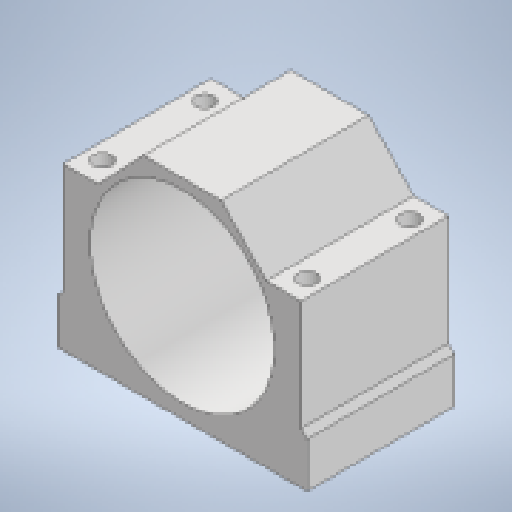
# Autodesk Inventor part: Spindle_Holder
Saved by Autodesk Inventor 2023 (Build 270158000, 158)
## iProperties
Created: 2022-05-06
Part Number: Spindle_Holder
Material: Generic
Document SubType Name: Modeling
Designer: plebbb
Density: 1 g/cm^3
Appearance: Default
Author: plebbb
Autodesk Inventor part; units mm, degrees
ref_plane "YZ Plane" through (0, 0, 0) normal (1, 0, 0) x (0, 1, 0)
ref_plane "XZ Plane" through (0, 0, 0) normal (0, 1, 0) x (-1, 0, 0)
ref_plane "XY Plane" through (0, 0, 0) normal (0, 0, 1) x (1, 0, 0)
sketch "Sketch1" plane through (0, 0, 0) normal (0, 0, 1) x (1, 0, 0)
  line L0 (0, 0) -> (122, 0)
  circle A0 centre (61, 52) radius 45
  line L1 (3, 78.943) -> (20, 78.943)
  line L2 (20, 78.943) -> (42, 102)
  line L3 (42, 102) -> (80, 102)
  line L4 (80, 102) -> (102, 78.943)
  line L5 (102, 78.943) -> (119, 78.943)
  line L6 (3, 25.057) -> (0, 22.057)
  line L7 (0, 22.057) -> (0, 0)
  line L8 (122, 0) -> (122, 22.057)
  line L9 (122, 22.057) -> (119, 25.057)
  line L10 (119, 25.057) -> (119, 78.943)
  line L11 (16, 52) -> (3, 52)
  line L12 (3, 52) -> (3, 25.057)
  line L13 (3, 52) -> (3, 78.943)
  point P0 (61, 0)
  point P1 (61, 102)
  dimension "d3" = 90
  dimension "d0" = 79
  dimension "d1" = 122
  dimension "d2" = 52
  dimension "d4" = 17
  dimension "d5" = 38
  dimension "d6" = 102
  dimension "d7" = 116
  dimension "d8" = 135
  constraints: 28 end point, 4 equal length, 4 horizontal, 4 vertical, 2 horizontal alignment, 2 midpoint, 2 vertical alignment, 1 collinear, 1 parallel, 1 perpendicular, 1 point on line, 2 other
  measures "d0" distance of L0.end L5.end
  measures "d1" distance of L0.start L0.end
  measures "d2" distance of point (61, 0) point (61, 52)
  measures "d4" distance of L4.end L5.end
  measures "d5" distance of L2.end L3.end
  measures "d6" distance from line of L0.end L3
  measures "d7" distance of L5.end L1.start
  measures "d8" angle of L7 L6
extrude "Extrusion1" add sketch "Sketch1" along normal blind 72
sketch "Sketch2" plane through (0, 0, 0) normal (0, -1, 0) x (1, 0, 0)
  line L0 (11, 11) -> (111, 11) construction
  line L1 (111, 11) -> (111, 61) construction
  line L2 (111, 61) -> (11, 61) construction
  line L3 (11, 61) -> (11, 11) construction
  circle A0 centre (11, 11) radius 4.5
  circle A1 centre (111, 11) radius 4.5
  circle A2 centre (111, 61) radius 4.5
  circle A3 centre (11, 61) radius 4.5
  line L4 (0, 72) -> (122, 72) construction
  line L5 (0, 0) -> (0, 72) construction
  point P0 (61, 61)
  point P1 (61, 72)
  point P2 (11, 36)
  point P3 (0, 36)
  dimension "d11" = 100
  dimension "d12" = 50
  dimension "d13" = 9
  constraints: 8 end point, 4 centre point, 4 coincident, 4 midpoint, 3 equal radius, 2 parallel, 1 horizontal, 1 horizontal alignment, 1 perpendicular, 1 vertical alignment
  measures "d11" distance of L1.end L2.end
  measures "d12" distance of L0.end L1.end
  measures "d13" diameter of A3
extrude "Extrusion2" cut sketch "Sketch2" against normal up to surface (78.943 mm away)
body "Solid1"
